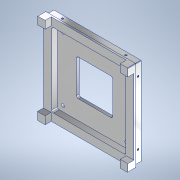
# Autodesk Inventor part: memesat top panel in progress
Saved by Autodesk Inventor 2022 (Build 260153000, 153)
## iProperties
Created: 2020-02-20
Part Number: memesat top panel in progress
Material: Aluminum 6061
Document SubType Name: Modeling
Designer: UGA SSRL
Density: 2.7 g/cm^3
Appearance: Aluminum - Flat
Mass: 57.0038 g
Surface Area: 222.367 cm^2
Volume: 21.1125 cm^3
Author: UGA SSRL
Autodesk Inventor part; units mm, degrees
ref_plane "YZ Plane" through (0, 0, 0) normal (1, 0, 0) x (0, 1, 0)
ref_plane "XZ Plane" through (0, 0, 0) normal (0, 1, 0) x (-1, 0, 0)
sketch "Sketch1" plane through (0, 0, 0) normal (0, 1, 0) x (-1, 0, 0)
  line L0 (50, 50) -> (-50, 50)
  line L1 (-50, 50) -> (-50, -50)
  line L2 (-50, -50) -> (50, -50)
  line L3 (50, -50) -> (50, 50)
  point P0 (0, 0)
  dimension "d0" = 100
  dimension "d1" = 100
  dimension "d2" = 50
  dimension "d3" = 50
  constraints: 8 end point, 2 parallel, 1 horizontal, 1 perpendicular
  measures "d0" distance of L2.end L1.end
  measures "d1" distance of L1.end L0.end
  measures "d2" distance from line of L3 point (0, 0)
  measures "d3" distance from line of L0 point (0, 0)
extrude "Extrusion1" add sketch "Sketch1" against normal blind 2
sketch "Sketch2" plane through (0, -2, 0) normal (0, -1, 0) x (1, 0, 0)
  line L0 (-50, 50) -> (-50, -50) projected
  line L1 (-50, 50) -> (-41.5, 50)
  line L2 (-41.5, 50) -> (-41.5, 41.5)
  line L3 (-41.5, 41.5) -> (-50, 41.5)
  line L4 (-50, 41.5) -> (-50, 50)
  line L5 (0, 0) -> (0, 12.5485) construction
  line L6 (0, 0) -> (11.2114, 0) construction
  line L7 (-50, -50) -> (-50, 50)
  line L8 (-50, -50) -> (-41.5, -50)
  line L9 (-41.5, -50) -> (-41.5, -41.5)
  line L10 (-41.5, -41.5) -> (-50, -41.5)
  line L11 (-50, -41.5) -> (-50, -50)
  line L12 (50, 50) -> (50, -50)
  line L13 (50, 50) -> (41.5, 50)
  line L14 (41.5, 50) -> (41.5, 41.5)
  line L15 (41.5, 41.5) -> (50, 41.5)
  line L16 (50, 41.5) -> (50, 50)
  line L17 (50, -50) -> (50, 50)
  line L18 (50, -50) -> (41.5, -50)
  line L19 (41.5, -50) -> (41.5, -41.5)
  line L20 (41.5, -41.5) -> (50, -41.5)
  line L21 (50, -41.5) -> (50, -50)
  dimension "d6" = 8.5
  dimension "d7" = 8.5
  constraints: 42 end point, 15 symmetric about line, 2 horizontal, 2 parallel, 1 perpendicular, 1 vertical
  measures "d6" distance of L2.end L3.end
  measures "d7" distance of L1.end L2.end
extrude "Extrusion2" add sketch "Sketch2" along normal blind 6.75
sketch "Sketch6" plane through (0, 0, 0) normal (0, 1, 0) x (1, 0, 0)
  line L0 (-50, 50) -> (-50, -50) projected
  line L1 (-50, -50) -> (50, -50) projected
  line L2 (50, 50) -> (-50, 50) projected
  line L3 (50, -50) -> (50, 50) projected
  line L4 (-48.5, -48.5) -> (-48.5, 48.5)
  line L5 (-48.5, 48.5) -> (48.5, 48.5)
  line L6 (48.5, 48.5) -> (48.5, -48.5)
  line L7 (48.5, -48.5) -> (-48.5, -48.5)
  line L8 (-46, 34.8675) -> (-46, -34.8675)
  line L9 (-37.725, -46) -> (37.8675, -46)
  line L10 (37.8675, 46) -> (-37.725, 46)
  line L11 (46, -32.465) -> (46, 31.195)
  line L12 (0, 0) -> (-0.6811, 0) construction
  line L13 (0, 0) -> (0, 0.5483) construction
  line L14 (-37.725, -46) -> (-46, -46)
  line L15 (-46, -46) -> (-46, -34.8675)
  line L16 (-46, 34.8675) -> (-46, 46)
  line L17 (-46, 46) -> (-37.725, 46)
  line L18 (37.8675, 46) -> (46, 46)
  line L19 (46, 46) -> (46, 31.195)
  line L20 (46, -32.465) -> (46, -46)
  line L21 (46, -46) -> (37.8675, -46)
  dimension "d80" = 1.5
  dimension "d81" = 2.5
  dimension "d161" = 2.5
  dimension "d162" = 2.5
  dimension "d173" = 2.5
  constraints: 36 end point, 2 collinear, 2 horizontal, 2 perpendicular, 2 point on line, 2 vertical, 3 other
  measures "d80" distance between parallel lines of L0 L4
  measures "d81" distance between parallel lines of L4 L8
  measures "d161" distance between parallel lines of L6 L11
  measures "d162" distance between parallel lines of L5 L10
  measures "d173" distance between parallel lines of L9 L7
extrude "Extrusion5" add sketch "Sketch6" along normal blind 7.5 contours L4 L5 L6 L7
ref_plane "Work Plane1" through (-50, 0, -50) normal (0.7071068, 0, -0.7071068) x (0, -1, 0)
fillet "Fillet3" radius 0.5 4 edges at (-50, -4.375, -50) (50, -4.375, -50) (50, -4.375, 50) (-50, -4.375, 50)
fillet "Fillet4" radius 0.5 8 edges at (-48.5, 3.75, -48.5) (-46, 3.75, -46) (46, 3.75, -46) (48.5, 3.75, -48.5) (48.5, 3.75, 48.5) (46, 3.75, 46) (-48.5, 3.75, 48.5) (-46, 3.75, 46)
sketch "Sketch31" plane through (0, 0, 0) normal (0, 1, 0) x (1, 0, 0)
  line L0 (-45.5, -46) -> (45.5, -46) projected
  arc A0 (45.5, -46) -> (46, -45.5) centre (45.5, -45.5) ccw projected
  line L1 (46, -45.5) -> (46, 45.5) projected
  arc A1 (46, 45.5) -> (45.5, 46) centre (45.5, 45.5) ccw projected
  line L2 (45.5, 46) -> (-45.5, 46) projected
  arc A2 (-45.5, 46) -> (-46, 45.5) centre (-45.5, 45.5) ccw projected
  line L3 (-46, 45.5) -> (-46, -45.5) projected
  line L4 (48, -48.5) -> (-48, -48.5) projected
  arc A3 (-48.5, -48) -> (-48, -48.5) centre (-48, -48) ccw projected
  line L5 (-48.5, -48) -> (-48.5, 48) projected
  arc A4 (-48, 48.5) -> (-48.5, 48) centre (-48, 48) ccw projected
  line L6 (-48, 48.5) -> (48, 48.5) projected
  arc A5 (48.5, 48) -> (48, 48.5) centre (48, 48) ccw projected
  line L7 (48.5, 48) -> (48.5, -48) projected
  arc A6 (48, -48.5) -> (48.5, -48) centre (48, -48) ccw projected
  arc A7 (-46, -45.5) -> (-45.5, -46) centre (-45.5, -45.5) ccw projected
  point P0 (0, 0)
extrude "Extrusion24" add sketch "Sketch31" along normal up to surface (7.5 mm away) contours A7 L3 A2 L2 A1 L1 A0 L0
sketch "Sketch32" plane through (48, 0, -48.5) normal (0, 0, -1) x (-1, 0, 0)
  circle A0 centre (13, 4) radius 1.727 projected
  circle A1 centre (83, 4) radius 1.727 projected
  point P0 (48, 0)
hole "Hole7" at (35, 4, -48.5) at (-35, 4, -48.5) direction (0, 0, 1) diameter 2.1565 depth 4 thread size "4-40 UNC" class "2B" standard "ANSI Unified Screw Threads"
pattern_circular "Circular Pattern1" count 4 over 360 about axis through (0, -10, 0) along (0, 1, 0) of "Hole7"
sketch "Sketch38" plane through (0, 7.5, 0) normal (0, 1, 0) x (1, 0, 0)
  arc A0 (-48.5, -48) -> (-48, -48.5) centre (-48, -48) ccw projected
  line L0 (-48, -48.5) -> (48, -48.5) projected
  arc A1 (48, -48.5) -> (48.5, -48) centre (48, -48) ccw projected
  line L1 (48.5, -48) -> (48.5, 48) projected
  arc A2 (48.5, 48) -> (48, 48.5) centre (48, 48) ccw projected
  line L2 (48, 48.5) -> (-48, 48.5) projected
  arc A3 (-48, 48.5) -> (-48.5, 48) centre (-48, 48) ccw projected
  line L3 (-48.5, 48) -> (-48.5, -48) projected
  line L4 (-40.5, -40.5) -> (40.5, -40.5)
  line L5 (40.5, -40.5) -> (40.5, 40.5)
  line L6 (40.5, 40.5) -> (-40.5, 40.5)
  line L7 (-40.5, 40.5) -> (-40.5, -40.5)
  point P0 (0, 0)
  dimension "d339" = 8
  constraints: 8 end point, 3 other
  measures "d339" distance between parallel lines of L3 L7
extrude "Extrusion29" cut sketch "Sketch38" against normal blind 5 contours L7 L6 L5 L4
sketch "Sketch40" plane through (0, -2, 0) normal (0, -1, 0) x (1, 0, 0)
  line L0 (-41, -41) -> (41, -41)
  line L1 (41, -41) -> (41, 41)
  line L2 (41, 41) -> (-41, 41)
  line L3 (-41, 41) -> (-41, -41)
  point P0 (0, 0)
  point P1 (0, 41)
  point P2 (-41, 0)
  dimension "d347" = 82
  dimension "d348" = 82
  constraints: 8 end point, 2 midpoint, 2 parallel, 1 horizontal, 1 horizontal alignment, 1 perpendicular, 1 vertical alignment
  measures "d347" distance of L2.end L1.end
  measures "d348" distance of L1.end L0.end
extrude "Extrusion31" cut sketch "Sketch40" against normal blind 1.5
fillet "Fillet13" radius 2 4 edges at (-41, -1.25, -41) (41, -1.25, -41) (41, -1.25, 41) (-41, -1.25, 41)
sketch "Sketch41" plane through (0, -0.5, 0) normal (0, -1, 0) x (1, 0, 0)
  line L0 (0, 0) -> (0, 14.4842) construction
  line L1 (0, 0) -> (-9.8024, 0) construction
  point P0 (-35, -35)
  point P1 (-35, 35)
  point P2 (35, -35)
  point P3 (35, 35)
  dimension "d352" = 35
  dimension "d353" = 35
  constraints: 4 end point, 3 symmetric about line, 1 horizontal, 1 vertical
  measures "d352" horizontal distance of L0.start point (-35, -35)
  measures "d353" horizontal distance of point (-35, -35) L0.start
hole "Hole9" at (-35, -0.5, -35) at (-35, -0.5, 35) at (35, -0.5, -35) at (35, -0.5, 35) direction (0, 1, 0) diameter 3.454 end through all clearance for "Flat Head Machine Screw (82)" size "#4" standard "Ansi Unified Screw Threads"
sketch "Sketch42" plane through (0, -0.5, 0) normal (0, -1, 0) x (1, 0, 0)
  line L0 (-20, -20) -> (20, -20)
  line L1 (20, -20) -> (20, 20)
  line L2 (20, 20) -> (-20, 20)
  line L3 (-20, 20) -> (-20, -20)
  point P0 (0, 0)
  point P1 (0, 20)
  point P2 (-20, 0)
  dimension "d361" = 40
  dimension "d362" = 40
  constraints: 8 end point, 2 midpoint, 2 parallel, 1 horizontal, 1 horizontal alignment, 1 perpendicular, 1 vertical alignment
  measures "d361" distance of L1.end L2.end
  measures "d362" distance of L2.end L0.start
extrude "Extrusion32" cut sketch "Sketch42" against normal through all
fillet "Fillet14" radius 2 4 edges at (-20, 1, -20) (-20, 1, 20) (20, 1, -20) (20, 1, 20)
sketch "Sketch43" plane through (0, 2.5, 0) normal (0, 1, 0) x (1, 0, 0)
  line L0 (18, -20) -> (-18, -20) projected
  arc A0 (-20, -18) -> (-18, -20) centre (-18, -18) ccw projected
  line L1 (-20, -18) -> (-20, 18) projected
  arc A1 (-18, 20) -> (-20, 18) centre (-18, 18) ccw projected
  line L2 (-18, 20) -> (18, 20) projected
  arc A2 (20, 18) -> (18, 20) centre (18, 18) ccw projected
  line L3 (20, 18) -> (20, -18) projected
  arc A3 (18, -20) -> (20, -18) centre (18, -18) ccw projected
  circle A4 centre (35, 35) radius 1.727 projected
  circle A5 centre (-35, 35) radius 1.727 projected
  circle A6 centre (-35, -35) radius 1.727 projected
  circle A7 centre (35, -35) radius 1.727 projected
  line L4 (40.5, 40.5) -> (40.5, -40.5) projected
  line L5 (-40.5, 40.5) -> (40.5, 40.5) projected
  line L6 (-40.5, -40.5) -> (-40.5, 40.5) projected
  line L7 (40.5, -40.5) -> (-40.5, -40.5) projected
  point P0 (0, 0)
extrude "Extrusion33" add sketch "Sketch43" along normal up to surface (5 mm away)
sketch "Sketch44" plane through (0, -0.5, 0) normal (0, -1, 0) x (1, 0, 0)
  line L0 (-18, 20) -> (18, 20) projected
  arc A0 (20, 18) -> (18, 20) centre (18, 18) ccw projected
  line L1 (20, 18) -> (20, -18) projected
  arc A1 (18, -20) -> (20, -18) centre (18, -18) ccw projected
  line L2 (18, -20) -> (-18, -20) projected
  arc A2 (-20, -18) -> (-18, -20) centre (-18, -18) ccw projected
  line L3 (-20, -18) -> (-20, 18) projected
  arc A3 (-18, 20) -> (-20, 18) centre (-18, 18) ccw projected
  circle A4 centre (35, -35) radius 1.727 projected
  circle A5 centre (-35, -35) radius 1.727 projected
  circle A6 centre (-35, 35) radius 1.727 projected
  circle A7 centre (35, 35) radius 1.727 projected
  arc A8 (-39, 41) -> (-41, 39) centre (-39, 39) ccw projected
  line L4 (-41, -39) -> (-41, 39) projected
  arc A9 (-41, -39) -> (-39, -41) centre (-39, -39) ccw projected
  line L5 (39, -41) -> (-39, -41) projected
  arc A10 (39, -41) -> (41, -39) centre (39, -39) ccw projected
  line L6 (41, 39) -> (41, -39) projected
  arc A11 (41, 39) -> (39, 41) centre (39, 39) ccw projected
  line L7 (-39, 41) -> (39, 41) projected
  point P0 (0, 0)
extrude "Extrusion34" cut sketch "Sketch44" against normal blind 5
equation "\"d2\" = 0.5 * d0"
equation "\"d3\" = 0.5 * d1"
equation "\"d33\" = 0.5 * d31"
equation "\"d36\" = 0.5 * d35"
equation "\"d31\" = 5"
equation "\"d35\" = 5"
body "Solid1"
